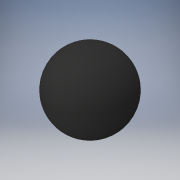
# Autodesk Inventor part: CapBall2
Saved by Autodesk Inventor 2017 (Build 210142000, 142)
## iProperties
Created: 2017-01-28
Part Number: CapBall2
Material: Rubber
Document SubType Name: Modeling
Designer: RoboticsUser
Density: 0.93 g/cm^3
Appearance: Rubber - Black
Mass: 73899.3 g
Surface Area: 8938.32 cm^2
Volume: 79461.7 cm^3
Author: RoboticsUser
Autodesk Inventor part; units mm, degrees
ref_plane "YZ Plane" through (0, 0, 0) normal (1, 0, 0) x (0, 1, 0)
ref_plane "XZ Plane" through (0, 0, 0) normal (0, 1, 0) x (-1, 0, 0)
ref_plane "XY Plane" through (0, 0, 0) normal (0, 0, 1) x (1, 0, 0)
sketch "Sketch1" plane through (0, 0, 0) normal (0, 0, 1) x (1, 0, 0)
  circle A0 centre (0, 0) radius 266.7
  line L0 (0, 266.7) -> (339.5925, 0)
  line L1 (339.5925, 0) -> (0, 0)
  line L2 (0, 0) -> (0, 266.7)
  dimension "d0" = 533.4
  dimension "d6" = 431.8008
  dimension "d7" = 266.7
  dimension "d8" = 339.5925
  constraints: 6 end point, 1 coincident, 1 horizontal, 1 vertical alignment, 2 other
  measures "d6" distance of L0.start L0.end
  measures "d7" distance of L1.end L0.start
  measures "d8" distance of L0.end L1.end
extrude "Extrusion1" add sketch "Sketch1" along normal mid plane 533.4 contours L2 L1 A0 | A0 L0 | L0 A0 L1 L2
fillet "Fillet1" radius 266.7 1 edges at (-266.7, 0, 266.7)
sketch "Sketch2" plane through (0, 0, -266.7) normal (0, 0, -1) x (-1, 0, 0)
  point P0 (0, 0)
fillet "Fillet2" radius 266.7 1 edges at (-266.7, 0, -266.7)
body "Solid1"
